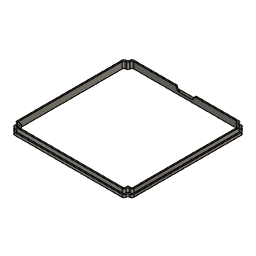
SolderingStation_BottomBevel (Autodesk Fusion 360 design; units mm, degrees)
Autodesk Fusion 360 part; units mm, degrees
sketch "Sketch1" plane through (0, 0, 0) normal (0, 0, 1) x (1, 0, 0)
  line L0 (45.1, 45.1) -> (-45.1, -45.1) construction
  line L1 (-45.1, 45.1) -> (45.1, -45.1) construction
  line L2 (45.1, 45.1) -> (45.1, 42) construction
  line L3 (45.1, 42) -> (42, 42)
  line L4 (42, 42) -> (42, 45.1)
  line L5 (-42, 42) -> (-45.1, 42)
  line L6 (-42, 45.1) -> (-42, 42)
  line L7 (-42, -42) -> (-42, -45.1)
  line L8 (-45.1, -42) -> (-42, -42)
  line L9 (42, -42) -> (45.1, -42)
  line L10 (42, -45.1) -> (42, -42)
  line L11 (-42, 45.1) -> (42, 45.1)
  line L12 (45.1, 42) -> (45.1, -42)
  line L13 (42, -45.1) -> (-42, -45.1)
  line L14 (-45.1, -42) -> (-45.1, 42)
  line L15 (43, 43) -> (43, 46.1)
  line L16 (-43, 46.1) -> (43, 46.1)
  line L17 (-43, 46.1) -> (-43, 43)
  line L18 (-43, 43) -> (-46.1, 43)
  line L19 (-46.1, -43) -> (-46.1, 43)
  line L20 (-46.1, -43) -> (-43, -43)
  line L21 (-43, -43) -> (-43, -46.1)
  line L22 (43, -46.1) -> (-43, -46.1)
  line L23 (43, -46.1) -> (43, -43)
  line L24 (43, -43) -> (46.1, -43)
  line L25 (46.1, 43) -> (46.1, -43)
  line L26 (46.1, 43) -> (43, 43)
  dimension "d1" = 90.2
  dimension "d2" = 90.2
  dimension "d3" = 3.1
  dimension "d5" = 360
  dimension "d6" = 1
  constraint coincident L0 origin
  constraint coincident L1 origin
  constraint coincident L0 L3.end
  constraint perpendicular L2 L3
  measures "d1" distance of L0.end L1.end
  measures "d2" distance of L1.start L0.end
  measures "d3" distance of L0.start L2.end
extrude "Extrude1" add sketch "Sketch1" along normal blind 5
fillet "Fillet1" radius 1.5 18 edges at (-43, 46.1, 2.5) (-43, 43, 2.5) (-46.1, 43, 2.5) (-42, 45.1, 2.5) (-42, 42, 2.5) (-45.1, 42, 2.5) (42, 45.1, 2.5) (42, 42, 2.5) (45.1, 42, 2.5) (43, 46.1, 2.5) (43, 43, 2.5) (46.1, 43, 2.5) (46.1, -43, 2.5) (43, -46.1, 2.5) (43, -43, 2.5) (-43, -43, 2.5) (-46.1, -43, 2.5) (-43, -46.1, 2.5)
sketch "Sketch2" plane through (0, 0, 0) normal (0, 0, 1) x (1, 0, 0)
  line L0 (-43, -46.1) -> (43, -46.1)
  line L1 (43, -46.1) -> (43, -43)
  line L2 (43, -43) -> (46.1, -43)
  line L3 (46.1, -43) -> (46.1, 43)
  line L4 (46.1, 43) -> (43, 43)
  line L5 (43, 43) -> (43, 46.1)
  line L6 (43, 46.1) -> (-43, 46.1)
  line L7 (-43, 46.1) -> (-43, 43)
  line L8 (-43, 43) -> (-46.1, 43)
  line L9 (-46.1, 43) -> (-46.1, -43)
  line L10 (-46.1, -43) -> (-43, -43)
  line L11 (-43, -43) -> (-43, -46.1)
  line L12 (44, -44) -> (47.1, -44)
  line L13 (47.1, -44) -> (47.1, 44)
  line L14 (47.1, 44) -> (44, 44)
  line L15 (44, 44) -> (44, 47.1)
  line L16 (44, 47.1) -> (-44, 47.1)
  line L17 (-44, 47.1) -> (-44, 44)
  line L18 (-44, 44) -> (-47.1, 44)
  line L19 (-47.1, 44) -> (-47.1, -44)
  line L20 (-47.1, -44) -> (-44, -44)
  line L21 (-44, -44) -> (-44, -47.1)
  line L22 (-44, -47.1) -> (44, -47.1)
  line L23 (44, -47.1) -> (44, -44)
  line L24 (45.1, 42) -> (42, 42)
  line L25 (42, 42) -> (42, 45.1)
  line L26 (42, 45.1) -> (-42, 45.1)
  line L27 (-42, 45.1) -> (-42, 42)
  line L28 (-42, 42) -> (-45.1, 42)
  line L29 (-45.1, 42) -> (-45.1, -42)
  line L30 (-45.1, -42) -> (-42, -42)
  line L31 (-42, -42) -> (-42, -45.1)
  line L32 (-42, -45.1) -> (42, -45.1)
  line L33 (42, -45.1) -> (42, -42)
  line L34 (42, -42) -> (45.1, -42)
  line L35 (45.1, -42) -> (45.1, 42)
  dimension "d11" = 1
  dimension "d16" = -1
  constraint horizontal L0
  constraint perpendicular L0 L1
  constraint perpendicular L1 L2
  constraint perpendicular L2 L3
  constraint perpendicular L3 L4
  constraint perpendicular L2 L5
  constraint perpendicular L3 L6
  constraint perpendicular L6 L7
  constraint perpendicular L7 L8
  constraint perpendicular L8 L9
  constraint perpendicular L9 L10
  constraint perpendicular L0 L11
extrude "Extrude2" add sketch "Sketch2" along normal blind 2 contours L0 L1 L2 L3 L4 L5 L6 L7 L8 L9 L10 L11 | L12 L13 L14 L15 L16 L17 L18 L19 L20 L21 L22 L23
fillet "Fillet2" radius 1.5 12 edges at (44, -47.1, 1) (44, -44, 1) (47.1, -44, 1) (47.1, 44, 1) (44, 44, 1) (44, 47.1, 1) (-44, 44, 1) (-44, 47.1, 1) (-47.1, 44, 1) (-44, -44, 1) (-47.1, -44, 1) (-44, -47.1, 1)
fillet "Fillet3" [suppressed]
fillet "Fillet4" radius 1.5 2 edges at (-42, 42, 1) (42, 42, 1)
sketch "Sketch3" plane through (0, 47.1, 0) normal (0, 1, 0) x (-1, 0, 0)
  line L0 (42.5, 0) -> (42.5, 2)
  line L1 (42.5, 2) -> (-42.5, 2)
  line L2 (-42.5, 2) -> (-42.5, 0)
  line L3 (-42.5, 0) -> (42.5, 0)
  line L4 (-7, 5) -> (7, 5)
  line L5 (7, 5) -> (7, 2)
  line L6 (7, 2) -> (-7, 2)
  line L7 (-7, 2) -> (-7, 5)
  line L8 (0, 0) -> (0, 5) construction
  dimension "d21" = 3
  dimension "d22" = 14
  dimension "d23" = 7
  constraint horizontal L4
  constraint vertical L5
  constraint horizontal L6
  constraint vertical L7
  constraint coincident L8.start origin
  constraint coincident L4 L8.end
  constraint perpendicular L4 L8
  measures "d21" distance of L4.end L5.end
  measures "d22" distance of L4.start L4.end
  measures "d23" distance of L7 L8
extrude "Extrude3" cut sketch "Sketch3" against normal blind 2 contours L1 L4 L5 L6 L7
fillet "Fillet5" radius 2 2 edges at (7, 45.6, 2) (-7, 45.6, 2)
fillet "Fillet6" radius 1 2 edges at (7, 45.6, 5) (-7, 45.6, 5)
